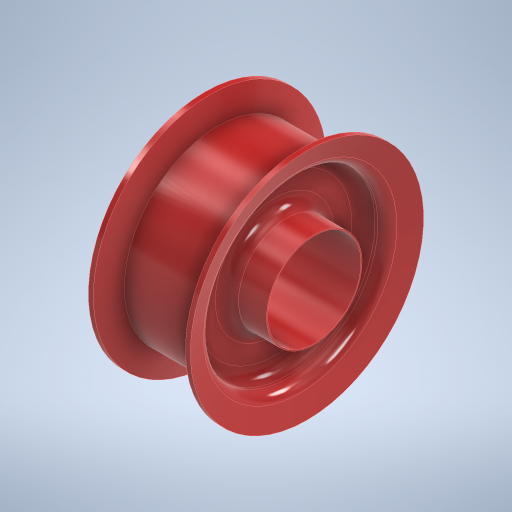
# Autodesk Inventor part: velg
Saved by Autodesk Inventor 2023 (Build 270158000, 158)
## iProperties
Created: 2023-08-28
Part Number: velg
Material: Steel, Alloy
Document SubType Name: Modeling
Designer: sigit
Density: 7.73 g/cm^3
Appearance: Red
Author: sigit
Autodesk Inventor part; units mm, degrees
ref_plane "XZ Plane" through (0, 0, 0) normal (0, 1, 0) x (-1, 0, 0)
ref_plane "XY Plane" through (0, 0, 0) normal (0, 0, 1) x (1, 0, 0)
sketch "Sketch1" plane through (0, 0, 0) normal (0, 0, 1) x (1, 0, 0)
  line L0 (-8, 38) -> (-17.8377, 38)
  line L1 (-17.8377, 38) -> (-21.8377, 50)
  line L2 (-19.7295, 50) -> (-21.8377, 50)
  line L3 (-19.7295, 50) -> (-16.3962, 40)
  line L4 (-16.3962, 40) -> (-2.5, 40)
  line L5 (-2.5, 40) -> (0, 40)
  line L6 (-8, 38) -> (-8, 0)
  line L7 (-8, 0) -> (0, 0)
  line L8 (8, 38) -> (17.8377, 38)
  line L9 (17.8377, 38) -> (21.8377, 50)
  line L10 (19.7295, 50) -> (21.8377, 50)
  line L11 (19.7295, 50) -> (16.3962, 40)
  line L12 (16.3962, 40) -> (2.5, 40)
  line L13 (2.5, 40) -> (0, 40)
  line L14 (8, 38) -> (8, 0)
  line L15 (8, 0) -> (0, 0)
  dimension "d14" = 2
  constraints: 32 end point, 1 horizontal, 1 vertical
  measures "d14" distance between parallel lines of L0 L4
ref_plane "Work Plane1" through (0, 0, 0) normal (1, 0, 0) x (0, 1, 0)
revolve "Revolution2" add sketch "Sketch1" angle 360 about axis through (-8, 0, 0) along (1, 0, 0)
fillet "Fillet1" radius 5 1 edges at (17.8377, -38, 0)
fillet "Fillet2" radius 5 1 edges at (-17.8377, -38, 0)
sketch "Sketch2" plane through (0, 0, 0) normal (1, 0, 0) x (0, 1, 0)
  circle A0 centre (0, 0) radius 20.5
  dimension "d11" = 41
  constraints: 1 centre point, 1 coincident
  measures "d11" diameter of A0
extrude "Extrusion1" add sketch "Sketch2" along normal mid plane 50
fillet "Fillet3" radius 5 4 edges at (-8, -38, 0) (-8, -20.5, 0) (8, -38, 0) (8, -20.5, 0)
sketch "Sketch3" plane through (0, 0, 0) normal (1, 0, 0) x (0, 1, 0)
  circle A0 centre (0, 0) radius 20
  dimension "d19" = 40
  constraints: 1 centre point, 1 coincident
  measures "d19" diameter of A0
extrude "Extrusion2" cut sketch "Sketch3" along normal mid plane 50
body "Solid1"
